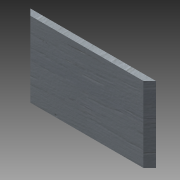
# Autodesk Inventor part: Aft_Support
Saved by Autodesk Inventor 2011 SP1 (Build 150282100, 282)
## iProperties
Created: 2011-06-12
Part Number: Aft_Support
Document SubType Name: Modeling
Designer: Andrew G. Meyer
Mass: 7.29736 g
Surface Area: 53.2198 cm^2
Volume: 7.29736 cm^3
Density: 1 g/cm^3
Author: Andrew G. Meyer
Autodesk Inventor part; units mm, degrees
ref_plane "YZ Plane" through (0, 0, 0) normal (1, 0, 0) x (0, 1, 0)
ref_plane "XZ Plane" through (0, 0, 0) normal (0, 1, 0) x (-1, 0, 0)
ref_plane "XY Plane" through (0, 0, 0) normal (0, 0, 1) x (1, 0, 0)
sketch "Sketch1" plane through (0, 0, 0) normal (0, 0, 1) x (1, 0, 0)
  line L0 (-19.4012, 18.8623) -> (44.0988, 18.8623)
  line L1 (44.0988, 18.8623) -> (44.0988, -19.2377)
  line L2 (44.0988, -19.2377) -> (-19.4012, -19.2377)
  line L3 (-19.4012, -19.2377) -> (-19.4012, 18.8623)
  point P0 (0, 0)
  dimension "d0" = 63.5
  dimension "d1" = 38.1
  constraints: 8 end point, 2 parallel, 1 horizontal, 1 perpendicular
  measures "d0" distance of L0.start L0.end
  measures "d1" distance of L2.end L0.start
extrude "Extrusion1" add sketch "Sketch1" along normal blind 3.175
chamfer "Chamfer1" distance 3.175 angle 45 2 edges at (44.0988, -0.1877, 3.175) (-19.4012, -0.1877, 3.175)
body "Solid1"
